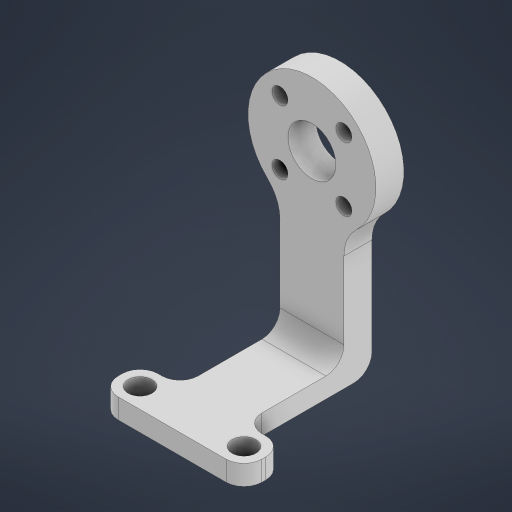
# Autodesk Inventor part: Bracket hinten
Saved by Autodesk Inventor 2023.2 (Build 272271000, 271)
## iProperties
Created: 2023-04-14
Part Number: Bracket hinten
Material: Generisch
Document SubType Name: Modeling
Designer: tadeus
Density: 1 g/cm^3
Appearance: Vorgabe
Author: tadeus
Autodesk Inventor part; units mm, degrees
ref_plane "YZ Plane" through (0, 0, 0) normal (1, 0, 0) x (0, 1, 0)
ref_plane "XZ Plane" through (0, 0, 0) normal (0, 1, 0) x (-1, 0, 0)
ref_plane "XY Plane" through (0, 0, 0) normal (0, 0, 1) x (1, 0, 0)
sketch "Skizze1" plane through (0, 0, 0) normal (0, 0, 1) x (1, 0, 0)
  line L0 (-12.5, 12.5) -> (12.5, 12.5) construction
  line L1 (12.5, 12.5) -> (12.5, -12.5) construction
  line L2 (12.5, -12.5) -> (-12.5, -12.5) construction
  line L3 (-12.5, -12.5) -> (-12.5, 12.5) construction
  line L4 (-12.5, 12.5) -> (12.5, -12.5) construction
  line L5 (12.5, 12.5) -> (-12.5, -12.5) construction
  circle A0 centre (-8, 8) radius 2
  line L6 (0, -16.0282) -> (0, 13.9718) construction
  line L7 (-17.9476, 0) -> (24.4038, 0) construction
  circle A1 centre (8, 8) radius 2
  circle A2 centre (-8, -8) radius 2
  circle A3 centre (8, -8) radius 2
  line L8 (-25, -47.5) -> (25, -47.5) construction
  arc A4 (8, -13.8564) -> (-8, -13.8564) centre (0, 0) ccw
  line L9 (-8, -8) -> (-8, -13.8564) construction
  line L10 (8, -8) -> (8, -13.8564) construction
  line L11 (-8, -13.8564) -> (-8, -47.5)
  line L12 (8, -13.8564) -> (8, -47.5)
  arc A5 (0, -16) -> (8, -13.8564) centre (0, 0) ccw construction
  arc A6 (-8, -13.8564) -> (0, -16) centre (0, 0) ccw construction
  line L13 (-8, -47.5) -> (8, -47.5)
  circle A7 centre (0, 0) radius 6
  line L14 (-8, -47.5) -> (8, -47.5)
  line L15 (8, -47.5) -> (8, -42.5)
  line L16 (8, -42.5) -> (-8, -42.5)
  line L17 (-8, -42.5) -> (-8, -47.5)
  line L18 (-8, -42.5) -> (-18, -42.5)
  line L19 (-18, -42.5) -> (-18, -47.5)
  line L20 (-18, -47.5) -> (-8, -47.5)
  line L21 (-8, -47.5) -> (-8, -42.5)
  line L22 (8, -42.5) -> (18, -42.5)
  line L23 (18, -42.5) -> (18, -47.5)
  line L24 (18, -47.5) -> (8, -47.5)
  line L25 (8, -47.5) -> (8, -42.5)
  point P0 (-8, -42.5)
  dimension "d0" = 25
  dimension "d1" = 25
  dimension "d2" = 4
  dimension "d4" = 8
  dimension "d5" = 8
  dimension "d8" = 16
  dimension "d11" = 16
  dimension "d14" = 50
  dimension "d15" = 47.5
  dimension "d16" = 32
  dimension "d17" = 25
  dimension "d20" = 12
  dimension "d21" = 5
  dimension "d22" = 10
  dimension "d23" = 10
  constraints: 52 end point, 8 centre point, 8 horizontal, 8 parallel, 8 perpendicular, 6 point on circle, 6 point on line, 3 vertical, 2 coincident, 2 midpoint, 1 collinear, 6 other
  measures "d0" distance of L1.end L2.end
  measures "d1" distance of L0.end L1.end
  measures "d2" diameter of A0
  measures "d4" distance from line of L6 A0.centre
  measures "d5" distance from line of L7 A0.centre
  measures "d8" distance of A0.centre A1.centre
  measures "d11" distance of A0.centre L9.start
  measures "d14" distance of L8.start L8.end
  measures "d15" distance from line of point (0, 0) L8
  measures "d16" diameter of A4
  measures "d17" distance from line of L6 L8.start
  measures "d20" diameter of A7
  measures "d21" distance of L15.end L14.end
  measures "d22" distance of L20.end L19.end
  measures "d23" distance of L23.end L24.end
extrude "Extrusion1" add sketch "Skizze1" along normal blind 7 contours L12 L16 L11 A4 | L12 L13 L11 L16
extrude "Extrusion2" add sketch "Skizze1" along normal blind 25 from surface at 7 contours L12 L13 L11 L16
extrude "Extrusion3" add sketch "Skizze1" along normal blind 10 from surface at 32 contours L22 L23 L24 L12 | L12 L13 L11 L16 | L11 L20 L19 L18
sketch "Skizze2" plane through (-8, -42.5, 7) normal (0, 1, 0) x (1, 0, 0)
  circle A0 centre (-5, -30) radius 3
  line L0 (-10, -35) -> (26, -35) projected
  line L1 (-10, -25) -> (-10, -35) projected
  point P0 (8, 7)
  dimension "d28" = 6
  dimension "d29" = 5
  dimension "d30" = 5
  constraints: 1 centre point
  measures "d28" diameter of A0
  measures "d29" distance from line of L0 A0.centre
  measures "d30" distance from line of L1 A0.centre
extrude "Extrusion4" cut sketch "Skizze2" against normal through all
mirror "Spiegeln1" about plane through (0, 0, 0) normal (1, 0, 0) of "Extrusion4"
fillet "Rundung1" radius 4.5 8 edges at (0, -47.5, 0) (-8, -45, 32) (-18, -45, 32) (-18, -45, 42) (18, -45, 42) (18, -45, 32) (8, -45, 32) (0, -42.5, 7)
fillet "Rundung2" radius 10 2 edges at (-8, -13.8564, 3.5) (8, -13.8564, 3.5)
